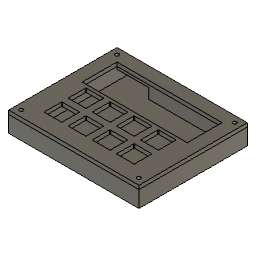
ZPad case (Autodesk Fusion 360 design; units mm, degrees)
part number: 2026-03-29-20-25-03-331
Autodesk Fusion 360 part; units mm, degrees
sketch "Sketch2" plane through (0, 0, 0) normal (0, 0, 1) x (1, 0, 0)
  line L0 (-31.2878, 30.0487) -> (51.6122, 30.0487)
  line L1 (51.6122, 30.0487) -> (51.6122, -35.5513)
  line L2 (51.6122, -35.5513) -> (-31.2878, -35.5513)
  line L3 (-31.2878, -35.5513) -> (-31.2878, 30.0487)
  line L4 (-41.2878, 40.0487) -> (61.6122, 40.0487)
  line L5 (61.6122, 40.0487) -> (61.6122, -45.5513)
  line L6 (61.6122, -45.5513) -> (-41.2878, -45.5513)
  line L7 (-41.2878, -45.5513) -> (-41.2878, 40.0487)
  circle A0 centre (-36.2878, 35.0487) radius 1.45
  circle A1 centre (56.6122, 35.0487) radius 1.45
  circle A2 centre (56.6122, -40.5513) radius 1.45
  circle A3 centre (-36.2878, -40.5513) radius 1.45
  line L8 (-25.3614, 0.0659) -> (-12.3614, 0.0659)
  line L9 (-25.3614, -13.9341) -> (-12.3614, -13.9341)
  line L10 (-25.8614, -0.4341) -> (-25.8614, -13.4341)
  line L11 (-11.8614, -0.4341) -> (-11.8614, -13.4341)
  arc A4 (-25.3614, 0.0659) -> (-25.8614, -0.4341) centre (-25.3614, -0.4341) ccw
  arc A5 (-11.8614, -0.4341) -> (-12.3614, 0.0659) centre (-12.3614, -0.4341) ccw
  arc A6 (-25.8614, -13.4341) -> (-25.3614, -13.9341) centre (-25.3614, -13.4341) ccw
  arc A7 (-12.3614, -13.9341) -> (-11.8614, -13.4341) centre (-12.3614, -13.4341) ccw
  line L12 (-6.3114, 0.0659) -> (6.6886, 0.0659)
  line L13 (-6.3114, -13.9341) -> (6.6886, -13.9341)
  line L14 (-6.8114, -0.4341) -> (-6.8114, -13.4341)
  line L15 (7.1886, -0.4341) -> (7.1886, -13.4341)
  arc A8 (-6.3114, 0.0659) -> (-6.8114, -0.4341) centre (-6.3114, -0.4341) ccw
  arc A9 (7.1886, -0.4341) -> (6.6886, 0.0659) centre (6.6886, -0.4341) ccw
  arc A10 (-6.8114, -13.4341) -> (-6.3114, -13.9341) centre (-6.3114, -13.4341) ccw
  arc A11 (6.6886, -13.9341) -> (7.1886, -13.4341) centre (6.6886, -13.4341) ccw
  line L16 (12.7386, 0.0659) -> (25.7386, 0.0659)
  line L17 (12.7386, -13.9341) -> (25.7386, -13.9341)
  line L18 (12.2386, -0.4341) -> (12.2386, -13.4341)
  line L19 (26.2386, -0.4341) -> (26.2386, -13.4341)
  arc A12 (12.7386, 0.0659) -> (12.2386, -0.4341) centre (12.7386, -0.4341) ccw
  arc A13 (26.2386, -0.4341) -> (25.7386, 0.0659) centre (25.7386, -0.4341) ccw
  arc A14 (12.2386, -13.4341) -> (12.7386, -13.9341) centre (12.7386, -13.4341) ccw
  arc A15 (25.7386, -13.9341) -> (26.2386, -13.4341) centre (25.7386, -13.4341) ccw
  line L20 (31.7886, 0.0659) -> (44.7886, 0.0659)
  line L21 (31.7886, -13.9341) -> (44.7886, -13.9341)
  line L22 (31.2886, -0.4341) -> (31.2886, -13.4341)
  line L23 (45.2886, -0.4341) -> (45.2886, -13.4341)
  arc A16 (31.7886, 0.0659) -> (31.2886, -0.4341) centre (31.7886, -0.4341) ccw
  arc A17 (45.2886, -0.4341) -> (44.7886, 0.0659) centre (44.7886, -0.4341) ccw
  arc A18 (31.2886, -13.4341) -> (31.7886, -13.9341) centre (31.7886, -13.4341) ccw
  arc A19 (44.7886, -13.9341) -> (45.2886, -13.4341) centre (44.7886, -13.4341) ccw
  line L24 (-25.3614, -18.9841) -> (-12.3614, -18.9841)
  line L25 (-25.3614, -32.9841) -> (-12.3614, -32.9841)
  line L26 (-25.8614, -19.4841) -> (-25.8614, -32.4841)
  line L27 (-11.8614, -19.4841) -> (-11.8614, -32.4841)
  arc A20 (-25.3614, -18.9841) -> (-25.8614, -19.4841) centre (-25.3614, -19.4841) ccw
  arc A21 (-11.8614, -19.4841) -> (-12.3614, -18.9841) centre (-12.3614, -19.4841) ccw
  arc A22 (-25.8614, -32.4841) -> (-25.3614, -32.9841) centre (-25.3614, -32.4841) ccw
  arc A23 (-12.3614, -32.9841) -> (-11.8614, -32.4841) centre (-12.3614, -32.4841) ccw
  line L28 (-6.3114, -18.9841) -> (6.6886, -18.9841)
  line L29 (-6.3114, -32.9841) -> (6.6886, -32.9841)
  line L30 (-6.8114, -19.4841) -> (-6.8114, -32.4841)
  line L31 (7.1886, -19.4841) -> (7.1886, -32.4841)
  arc A24 (-6.3114, -18.9841) -> (-6.8114, -19.4841) centre (-6.3114, -19.4841) ccw
  arc A25 (7.1886, -19.4841) -> (6.6886, -18.9841) centre (6.6886, -19.4841) ccw
  arc A26 (-6.8114, -32.4841) -> (-6.3114, -32.9841) centre (-6.3114, -32.4841) ccw
  arc A27 (6.6886, -32.9841) -> (7.1886, -32.4841) centre (6.6886, -32.4841) ccw
  line L32 (12.7386, -18.9841) -> (25.7386, -18.9841)
  line L33 (12.7386, -32.9841) -> (25.7386, -32.9841)
  line L34 (12.2386, -19.4841) -> (12.2386, -32.4841)
  line L35 (26.2386, -19.4841) -> (26.2386, -32.4841)
  arc A28 (12.7386, -18.9841) -> (12.2386, -19.4841) centre (12.7386, -19.4841) ccw
  arc A29 (26.2386, -19.4841) -> (25.7386, -18.9841) centre (25.7386, -19.4841) ccw
  arc A30 (12.2386, -32.4841) -> (12.7386, -32.9841) centre (12.7386, -32.4841) ccw
  arc A31 (25.7386, -32.9841) -> (26.2386, -32.4841) centre (25.7386, -32.4841) ccw
  line L36 (31.7886, -18.9841) -> (44.7886, -18.9841)
  line L37 (31.7886, -32.9841) -> (44.7886, -32.9841)
  line L38 (31.2886, -19.4841) -> (31.2886, -32.4841)
  line L39 (45.2886, -19.4841) -> (45.2886, -32.4841)
  arc A32 (31.7886, -18.9841) -> (31.2886, -19.4841) centre (31.7886, -19.4841) ccw
  arc A33 (45.2886, -19.4841) -> (44.7886, -18.9841) centre (44.7886, -19.4841) ccw
  arc A34 (31.2886, -32.4841) -> (31.7886, -32.9841) centre (31.7886, -32.4841) ccw
  arc A35 (44.7886, -32.9841) -> (45.2886, -32.4841) centre (44.7886, -32.4841) ccw
  line L40 (-28.3864, -35.5091) -> (47.8136, -35.5091)
  line L41 (-28.3864, 2.5909) -> (47.8136, 2.5909)
  line L42 (-28.3864, -35.5091) -> (-28.3864, 2.5909)
  line L43 (47.8136, -35.5091) -> (47.8136, 2.5909)
  line L44 (-31.2878, 30.0487) -> (51.6122, 30.0487)
  line L45 (51.6122, 30.0487) -> (51.6122, 2.5909)
  line L46 (51.6122, 2.5909) -> (-31.2878, 2.5909)
  line L47 (-31.2878, 2.5909) -> (-31.2878, 30.0487)
  line L48 (-31.2878, 30.0487) -> (-6.2878, 30.0487)
  line L49 (-6.2878, 30.0487) -> (-6.2878, 40.0487)
  line L50 (-6.2878, 40.0487) -> (-31.2878, 40.0487)
  line L51 (-31.2878, 40.0487) -> (-31.2878, 30.0487)
  dimension "d3" = 65.6
  dimension "d4" = 82.9
  dimension "d5" = 10
  dimension "d6" = 10
  dimension "d7" = 10
  dimension "d8" = 10
  dimension "d9" = 2.9
  dimension "d10" = 5
  dimension "d11" = 5
  dimension "d12" = 2.9
  dimension "d13" = 5
  dimension "d14" = 5
  dimension "d15" = 2.9
  dimension "d16" = 5
  dimension "d17" = 5
  dimension "d18" = 2.9
  dimension "d19" = 5
  dimension "d20" = 5
  dimension "d32" = 25
  constraint horizontal L0
  constraint vertical L1
  constraint horizontal L2
  constraint vertical L3
  constraint horizontal L4
  constraint vertical L5
  constraint horizontal L6
  constraint vertical L7
  constraint vertical L42
  constraint horizontal L44
  constraint vertical L45
  constraint horizontal L46
  constraint vertical L47
  constraint coincident L1 L45.end
  constraint horizontal L48
  constraint vertical L49
  constraint horizontal L50
  constraint vertical L51
  measures "d3" distance of L0.start L2.end
  measures "d4" distance of L1 L3
  measures "d5" distance of L1 L5
  measures "d6" distance of L3 L7
  measures "d7" distance of L0 L4
  measures "d8" distance of L2 L6
  measures "d9" diameter of A0
  measures "d10" distance of L7 A0.centre
  measures "d11" distance of L4 A0.centre
  measures "d12" diameter of A1
  measures "d13" distance of L4 A1.centre
  measures "d14" distance of L5 A1.centre
  measures "d15" diameter of A2
  measures "d16" distance of L5 A2.centre
  measures "d17" distance of L6 A2.centre
  measures "d18" diameter of A3
  measures "d19" distance of L7 A3.centre
  measures "d20" distance of L6 A3.centre
  measures "d32" distance of L0.start L48.end
extrude "Extrude1" add sketch "Sketch2" along normal blind 3 contours L0 L4 L44 L48 L49 L50 L51 | L0 L1 L3 L41 L44 L45 L46 L47 L48 | L0 L1 L2 L3 L4 L5 L6 L7 L44 L45 L47 L49 L51 | L1 L2 L3 L40 L42 L43 L46 | L40 L41 L42 L43 L46 | L8 L9 L10 L11 A4 A5 A6 A7 | L12 L13 L14 L15 A8 A9 A10 A11 | L16 L17 L18 L19 A12 A13 A14 A15 | L20 L21 L22 L23 A16 A17 A18 A19 | L24 L25 L26 L27 A20 A21 A22 A23 | L28 L29 L30 L31 A24 A25 A26 A27 | L32 L33 L34 L35 A28 A29 A30 A31 | L36 L37 L38 L39 A32 A33 A34 A35 makes body 1
extrude "Extrude2" add sketch "Sketch2" along normal blind 10 from surface at 3 contours L0 L4 L44 L48 L49 L50 L51 | L0 L1 L2 L3 L4 L5 L6 L7 L44 L45 L47 L49 L51 bodies 1
extrude "Extrude3" add sketch "Sketch2" along normal blind 3 from surface at 13 separate body makes body 2
extrude "Extrude4" add sketch "Sketch2" along normal blind 3 from surface at 13 separate body contours L0 L1 L3 L41 L44 L45 L46 L47 L48 makes body 3
combine "Combine1" operation cut target body 2 tool bodies 3
extrude "Extrude5" add sketch "Sketch2" along normal blind 8 from surface at 3 separate body contours L0 L4 L44 L48 L49 L50 L51 makes body 4
combine "Combine2" operation cut target body 1 tool bodies 4
